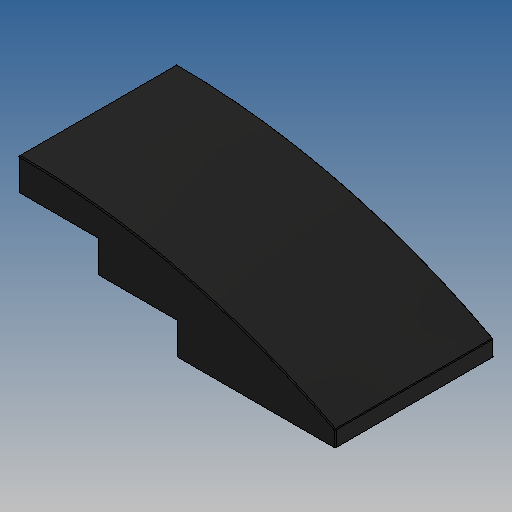
# Autodesk Inventor part: 93606-Black
Saved by Autodesk Inventor 2025 (Build 290162010, 162A)
## iProperties
Created: 2014-06-03
Part Number: 93606-Black
Material: ABS Plastic
Document SubType Name: Modeling
Designer: D. Kohfeld
Density: 1.06 g/cm^3
Appearance: Black
Mass: 1.59534 g
Surface Area: 21.0911 cm^2
Volume: 1.50504 cm^3
Author: D. Kohfeld
Autodesk Inventor part; units mm, degrees
ref_plane "YZ Plane" through (0, 0, 0) normal (1, 0, 0) x (0, 1, 0)
ref_plane "XZ Plane" through (0, 0, 0) normal (0, 1, 0) x (-1, 0, 0)
ref_plane "XY Plane" through (0, 0, 0) normal (0, 0, 1) x (1, 0, 0)
sketch "Sketch2" plane through (0, 0, 0) normal (0, 1, 0) x (-1, 0, 0)
  line L0 (-16, 8) -> (16, 8)
  line L1 (16, 8) -> (16, -8)
  line L2 (16, -8) -> (-16, -8)
  line L3 (-16, -8) -> (-16, 8)
  point P0 (0, 0)
  point P1 (0, 8)
  point P2 (-16, 0)
  dimension "d0" = 32
  dimension "d1" = 16
  constraints: 8 end point, 2 midpoint, 2 parallel, 1 horizontal, 1 horizontal alignment, 1 perpendicular, 1 vertical alignment
  measures "d0" distance of L1.end L2.end
  measures "d1" distance of L2.end L0.start
extrude "Extrusion1" add sketch "Sketch2" along normal blind 9.6
sketch "Sketch10" plane through (0, 0, 0) normal (0, 0, 1) x (1, 0, 0)
  line L0 (-16, 9.6) -> (16, 9.6) projected
  line L1 (-16, 0) -> (-16, 9.6) projected
  arc A0 (16, 1.6) -> (-16, 9.6) centre (-16, -58.4) ccw
  line L2 (16, 1.6) -> (16, 9.6)
  line L3 (-16, 0) -> (16, 0) projected
  line L4 (14.4, 0) -> (14.4, 1.6)
  line L5 (14.4, 1.6) -> (12.4422, 1.6)
  line L6 (-8, 3.2) -> (-8, 7.5163)
  line L7 (-6.4, 7.3024) -> (-6.4, 3.2)
  arc A1 (12.4422, 1.6) -> (-6.4, 7.3024) centre (-16, -58.4) ccw
  arc A2 (-8, 7.5163) -> (-14.4, 7.9807) centre (-16, -58.4) ccw
  line L8 (-14.4, 7.9807) -> (-14.4, 6.4)
  line L9 (1.6, 5.625) -> (1.6, 0)
  line L10 (0, 6.0435) -> (0, 0)
  line L11 (0, 3.2) -> (-6.4, 3.2)
  line L12 (-8, 6.4) -> (-14.4, 6.4)
  line L13 (-14.4, 6.4) -> (-16, 6.4)
  line L14 (16, 0) -> (16, 9.6) projected
  line L15 (1.6, 0) -> (14.4, 0)
  line L16 (0, 0) -> (-16, 0)
  line L17 (-16, 0) -> (-16, 6.4)
  line L18 (-6.4, 3.2) -> (-8, 3.2)
  dimension "d100" = 1.6
  dimension "d104" = 1.6
  dimension "d105" = 1.6
  dimension "d107" = 1.6
  dimension "d108" = 1.6
  dimension "d113" = 6.4
  dimension "d114" = 3.2
  dimension "d115" = 16
  dimension "d116" = 1.6
  constraints: 30 end point, 8 perpendicular, 8 point on circle, 5 point on line, 4 parallel, 3 centre point, 3 collinear, 2 concentric, 1 midpoint, 1 tangent
  measures "d100" distance from line of L2.start L3
  measures "d104" distance from line of L4 L3.end
  measures "d105" distance between parallel lines of L5 L3
  measures "d107" radial gap between concentric circles of A0 A2
  measures "d108" distance between parallel lines of L1 L8
  measures "d113" distance between parallel lines of L13 L3
  measures "d114" distance between parallel lines of L11 L3
  measures "d115" distance between parallel lines of L14 L10
  measures "d116" distance between parallel lines of L10 L9
extrude "Extrusion7" cut sketch "Sketch10" along normal through all both and the other way through all contours L0 L2 A0 | L13 L12 L6 L18 L11 L10 L3 L1
extrude "Extrusion8" cut sketch "Sketch10" along normal mid plane 12.8 contours L8 A2 L6 L12 | L3 L9 A1 L5 L4 | L11 L7 A1 L10
sketch "Sketch3" plane through (0, 0, 0) normal (0, -1, 0) x (1, 0, 0)
  circle A0 centre (12, 4) radius 2.4 construction
  line L0 (14.4, -6.4) -> (1.6, -6.4) projected
  line L1 (1.6, -6.4) -> (1.6, 6.4) projected
  line L2 (1.6, 6.4) -> (14.4, 6.4) projected
  line L3 (14.4, 6.4) -> (14.4, -6.4) projected
  circle A1 centre (8, 0) radius 3.2569
  circle A2 centre (8, 0) radius 2.4
  circle A3 centre (12, -4) radius 2.4 construction
  point P0 (8, 6.4)
  point P1 (1.6, 0)
  dimension "d97" = 4.8
  constraints: 6 tangent, 4 centre point, 2 midpoint, 1 coincident, 1 equal radius, 1 horizontal alignment, 1 vertical alignment
  measures "d97" diameter of A0
extrude "Extrusion2" add sketch "Sketch3" against normal up to next contours A1
sketch "Sketch11" plane through (-8, 3.2, 8) normal (0, -1, 0) x (1, 0, 0)
  line L0 (8, -1.6) -> (8, 0) projected
  line L1 (8, -14.4) -> (1.6, -14.4) projected
  line L2 (1.6, -14.4) -> (1.6, -1.6) projected
  circle A0 centre (4, -12) radius 2.4 construction
  line L3 (8, -11.4) -> (6.4, -11.4)
  line L4 (6.4, -11.4) -> (6.4, -12.6)
  line L5 (6.4, -12.6) -> (8, -12.6)
  line L6 (8, -11.4) -> (8, -12.6)
  line L7 (1.6, -1.6) -> (8, -1.6) projected
  circle A1 centre (4, -4) radius 2.4 construction
  line L8 (8, -4.6) -> (6.4, -4.6)
  line L9 (6.4, -4.6) -> (6.4, -3.4)
  line L10 (6.4, -3.4) -> (8, -3.4)
  line L11 (8, -3.4) -> (8, -4.6)
  circle A2 centre (4, -8) radius 1.6
  line L12 (6.4, -7.4) -> (8, -7.4)
  line L13 (8, -7.4) -> (8, -8.6)
  line L14 (8, -8.6) -> (6.4, -8.6)
  line L15 (6.4, -8.6) -> (6.4, -7.4)
  point P0 (8, -8)
  point P1 (6.4, -12)
  point P2 (6.4, -4)
  point P3 (6.4, -8)
  dimension "d119" = 1.2
  dimension "d129" = 4.8
  constraints: 24 end point, 8 tangent, 5 parallel, 5 perpendicular, 4 vertical alignment, 3 centre point, 3 equal length, 3 horizontal alignment, 3 midpoint, 2 horizontal, 1 collinear, 1 equal radius
  measures "d119" distance of L3.end L4.end
  measures "d129" diameter of A0
extrude "Extrusion9" add sketch "Sketch11" against normal up to next
sketch "Sketch12" plane through (-16, 6.4, 8) normal (0, -1, 0) x (1, 0, 0)
  line L0 (1.6, -1.6) -> (8, -1.6) projected
  line L1 (8, -14.4) -> (1.6, -14.4) projected
  line L2 (1.6, -14.4) -> (1.6, -1.6) projected
  line L3 (8, -3.4) -> (6.4, -3.4)
  line L4 (6.4, -3.4) -> (6.4, -4.6)
  line L5 (6.4, -4.6) -> (8, -4.6)
  line L6 (8, -4.6) -> (8, -3.4)
  circle A0 centre (4, -4) radius 2.4 construction
  circle A1 centre (4, -12) radius 2.4 construction
  line L7 (8, -11.4) -> (6.4, -11.4)
  line L8 (6.4, -11.4) -> (6.4, -12.6)
  line L9 (6.4, -12.6) -> (8, -12.6)
  line L10 (8, -12.6) -> (8, -11.4)
  line L11 (8, -7.4) -> (6.4, -7.4)
  line L12 (6.4, -7.4) -> (6.4, -8.6)
  line L13 (6.4, -8.6) -> (8, -8.6)
  line L14 (8, -8.6) -> (8, -7.4)
  circle A2 centre (4, -8) radius 1.6
  point P0 (16, -8)
  point P1 (6.4, -4)
  point P2 (6.4, -12)
  point P3 (6.4, -8)
  dimension "d122" = 1.2
  dimension "d130" = 4.8
  constraints: 24 end point, 8 tangent, 6 parallel, 4 equal length, 3 centre point, 3 horizontal, 3 horizontal alignment, 3 midpoint, 3 perpendicular, 3 vertical alignment, 1 equal radius
  measures "d122" distance between parallel lines of L3 L5
  measures "d130" diameter of A0
extrude "Extrusion10" add sketch "Sketch12" against normal up to next
fillet "Fillet1" radius 0.1 12 edges at (-16, 8, 8) (-16, 9.6, 0) (16, 0.8, 8) (16, 0.8, -8) (-16, 8, -8) (0.4924, 7.5697, 8) (0.4924, 7.5697, -8) (16, 1.6, 0) (-8, 4.8, 8) (0, 1.6, 8) (0, 1.6, -8) (-8, 4.8, -8)
equation "\"d4\" = lh"
equation "\"d100\" = wall"
equation "\"d104\" = wall"
equation "\"d105\" = 0.333333 * lh - topthk"
equation "\"d107\" = topthk"
equation "\"d108\" = d104"
equation "\"d113\" = 0.666667 * lh"
equation "\"d114\" = 0.333333 * lh"
equation "\"d115\" = 2 * lu"
equation "\"d116\" = wall"
equation "\"d109\" = 2 * lu - 2 * wall"
equation "\"d97\" = kd"
equation "\"d129\" = kd"
equation "\"lh\" = 9.6"
equation "\"wall\" = 1.6"
equation "\"topthk\" = 1.6"
equation "\"lu\" = 8"
equation "\"kd\" = 4.8"
body "Solid1"
